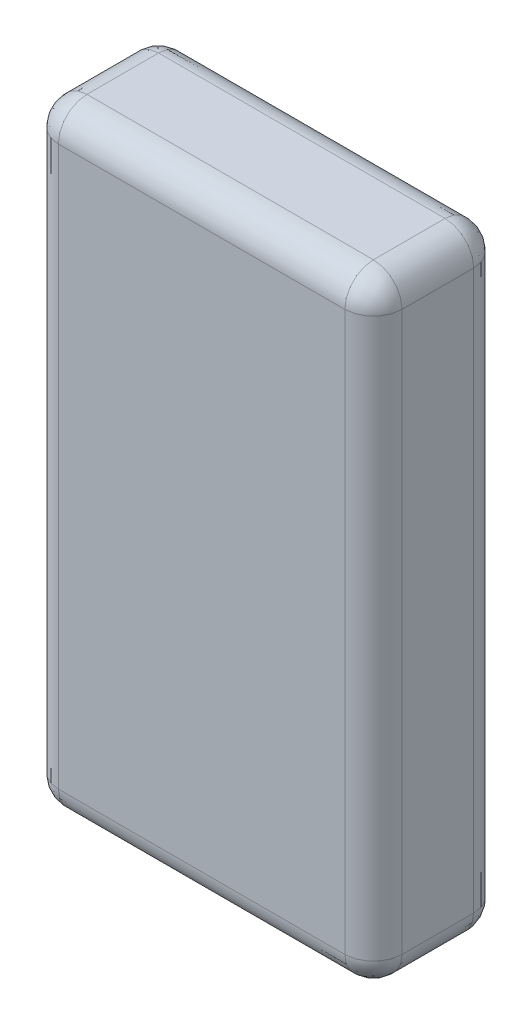
# Autodesk Inventor part: battery
Saved by Autodesk Inventor 2017 (Build 210142000, 142)
## iProperties
Created: 2017-04-29
Part Number: battery
Material: Generic
Document SubType Name: Modeling
Designer: X220T
Density: 1 g/cm^3
Appearance: Default
Author: X220T
Autodesk Inventor part; units mm, degrees
ref_plane "YZ Plane" through (0, 0, 0) normal (1, 0, 0) x (0, 1, 0)
ref_plane "XZ Plane" through (0, 0, 0) normal (0, 1, 0) x (-1, 0, 0)
ref_plane "XY Plane" through (0, 0, 0) normal (0, 0, 1) x (1, 0, 0)
sketch "Sketch1" plane through (0, 0, 0) normal (0, 0, 1) x (1, 0, 0)
  line L0 (-12, -21.5) -> (12, -21.5)
  line L1 (12, -21.5) -> (12, 21.5)
  line L2 (12, 21.5) -> (-12, 21.5)
  line L3 (-12, 21.5) -> (-12, -21.5)
  line L4 (-12, -21.5) -> (12, 21.5) construction
  line L5 (12, -21.5) -> (-12, 21.5) construction
  point P0 (0, 0)
  dimension "d0" = 24
  dimension "d1" = 43
  constraints: 12 end point, 2 midpoint, 2 parallel, 1 horizontal, 1 perpendicular
  measures "d0" distance of L1.end L2.end
  measures "d1" distance of L0.end L1.end
extrude "Extrusion1" add sketch "Sketch1" along normal mid plane 9
fillet "Fillet1" radius 2 12 edges at (0, 21.5, 4.5) (0, 21.5, -4.5) (12, 0, 4.5) (12, 0, -4.5) (12, 21.5, 0) (-12, 21.5, 0) (-12, 0, 4.5) (-12, 0, -4.5) (-12, -21.5, 0) (0, -21.5, 4.5) (0, -21.5, -4.5) (12, -21.5, 0)
body "Solid1"
